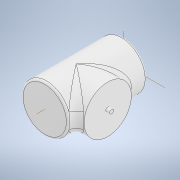
# Autodesk Inventor part: Link1
Saved by Autodesk Inventor 2021 (Build 250183000, 183)
## iProperties
Created: 2021-03-25
Part Number: Link1
Material: ABS 플라스틱
Document SubType Name: Modeling
Designer: jglee
Density: 1.06 g/cm^3
Appearance: 매끄러움 - 흰색
Mass: 2755.26 g
Surface Area: 1086.37 cm^2
Volume: 2599.3 cm^3
Author: jglee
Autodesk Inventor part; units mm, degrees
ref_plane "YZ Plane" through (0, 0, 0) normal (1, 0, 0) x (0, 1, 0)
ref_plane "XZ Plane" through (0, 0, 0) normal (0, 1, 0) x (-1, 0, 0)
ref_plane "XY Plane" through (0, 0, 0) normal (0, 0, 1) x (1, 0, 0)
sketch "스케치1" plane through (0, 0, 0) normal (0, 0, 1) x (1, 0, 0)
  circle A0 centre (0, 0) radius 60
  dimension "d0" = 120
  constraints: 1 centre point, 1 coincident
  measures "d0" diameter of A0
extrude "돌출1" add sketch "스케치1" along normal blind 200
fillet "모깎기1" radius 5 2 edges at (-60, 0, 0) (-60, 0, 200)
sketch "스케치2" plane through (0, 0, 0) normal (0, 0, -1) x (-1, 0, 0)
  circle A0 centre (0, 0) radius 5
  dimension "d4" = 10
  constraints: 1 centre point, 1 coincident
  measures "d4" diameter of A0
extrude "돌출2" cut sketch "스케치2" against normal blind 10
sketch "스케치3" plane through (0, 0, 0) normal (1, 0, 0) x (0, 1, 0)
  line L0 (-60, 5) -> (60, 5) projected
  line L1 (60, 195) -> (-60, 195) projected
  circle A0 centre (0, 120) radius 60
  point P0 (0, 0)
  dimension "d7" = 120
  dimension "d8" = 120
  constraints: 1 centre point
  measures "d7" diameter of A0
  measures "d8" distance of point (0, 0) A0.centre
extrude "돌출3" add sketch "스케치3" along normal blind 80
fillet "모깎기2" radius 20 4 edges at (42.4264, 42.4264, 162.4264) (42.4264, -42.4264, 162.4264) (42.4264, -42.4264, 77.5736) (42.4264, 42.4264, 77.5736)
sketch "스케치4" plane through (80, 0, 120) normal (1, 0, 0) x (0, 0, -1)
  circle A0 centre (0, 0) radius 5
  point P0 (120, 0)
  dimension "d12" = 10
  constraints: 1 centre point
  measures "d12" diameter of A0
extrude "돌출4" add sketch "스케치4" along normal blind 10
